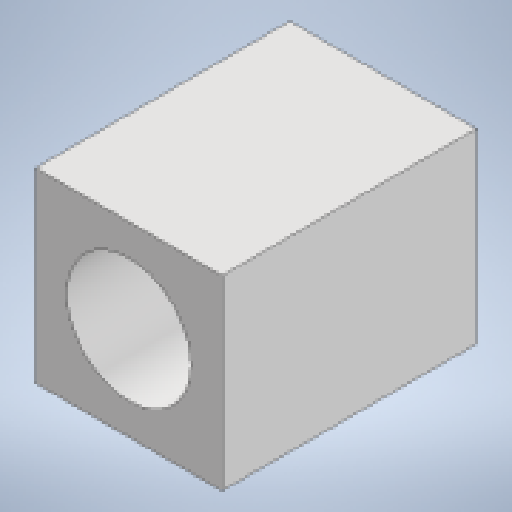
# Autodesk Inventor part: Brazo catapulta
Saved by Autodesk Inventor 2024 (Build 280153000, 153)
## iProperties
Created: 2025-03-01
Part Number: Brazo catapulta
Material: Genérico
Document SubType Name: Modeling
Designer: sergi
Density: 1 g/cm^3
Appearance: Valor por defecto
Author: sergi
Autodesk Inventor part; units mm, degrees
ref_plane "YZ Plane" through (0, 0, 0) normal (1, 0, 0) x (0, 1, 0)
ref_plane "XZ Plane" through (0, 0, 0) normal (0, 1, 0) x (-1, 0, 0)
ref_plane "XY Plane" through (0, 0, 0) normal (0, 0, 1) x (1, 0, 0)
sketch "Boceto1" plane through (0, 0, 0) normal (0, 1, 0) x (-1, 0, 0)
  line L0 (0, 0) -> (22, 0)
  line L1 (22, 0) -> (22, 30)
  line L2 (22, 30) -> (0, 30)
  line L3 (0, 30) -> (0, 0)
  dimension "d0" = 22
  dimension "d1" = 30
  constraints: 8 end point, 2 parallel, 1 horizontal, 1 perpendicular
  measures "d0" distance of L2.end L1.end
  measures "d1" distance of L1.end L0.end
extrude "Extrusión1" add sketch "Boceto1" along normal blind 22
sketch "Boceto2" plane through (-22, 0, 30) normal (0, 0, 1) x (1, 0, 0)
  line L0 (0, 0) -> (22, 0) projected
  line L1 (22, 0) -> (22, 22) projected
  line L2 (0, 22) -> (22, 22) projected
  line L3 (0, 0) -> (0, 22) projected
  line L4 (22, 22) -> (0, 0)
  circle A0 centre (11, 11) radius 7.3
  dimension "d4" = 14.6
  constraints: 2 end point, 1 centre point, 1 midpoint
  measures "d4" diameter of A0
extrude "Extrusión2" cut sketch "Boceto2" against normal through all contours A0 L4 | L4 A0
chamfer "Chaflán1" distance 6.5 angle 45 2 edges at (0, 22, 15) (0, 0, 15)
sketch "Boceto3" plane through (-22, 0, 30) normal (0, 0, 1) x (1, 0, 0)
  line L0 (-84.9, -39.92) -> (20.1, -39.92) projected
  line L1 (20.1, -39.92) -> (20.1, -9.92) projected
  line L2 (-84.9, -9.92) -> (20.1, -9.92) projected
  line L3 (-84.9, -39.92) -> (-84.9, -9.92) projected
  line L4 (0, 0) -> (-84.9, 0)
  line L5 (-88.7564, 6.9) -> (-92.3631, 6.9) projected
  line L6 (-84.9, 0) -> (-84.9, 4)
  line L7 (-84.9, 4) -> (-18.9, 4)
  line L8 (-18.9, 4) -> (0, 22)
  line L9 (22, 6.5) -> (15.5, 0) projected
  line L10 (22, 6.5) -> (22, 15.5) projected
  line L11 (15.5, 22) -> (22, 15.5) projected
  line L12 (0, 22) -> (15.5, 22) projected
  line L13 (0, 0) -> (0, 22) projected
  line L14 (0, 0) -> (15.5, 0) projected
  circle A0 centre (11, 11) radius 7.3 projected
  point P0 (22, 0)
  dimension "d10" = 4
  dimension "d11" = 66
  constraints: 8 end point, 2 horizontal, 1 vertical
  measures "d10" distance of L4.end L6.end
  measures "d11" distance of L6.end L7.end
extrude "Extrusión3" add sketch "Boceto3" against normal up to surface (30 mm away) contours L4 L6 L7 L8 L13
